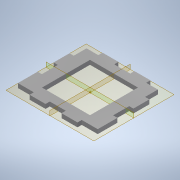
# Autodesk Inventor part: Plaat achter
Saved by Autodesk Inventor 2021 (Build 250183000, 183)
## iProperties
Manager: PJ / DCS
Company: Emmaüs Bovenbouw Aalter
Created: 2021-01-09
Part Number: Plaat achter
Material: S235
Catalog Web Link: http://emmausbovenbouw.op-weg.be/
Vendor: Emmaüsinstituut Bovenbouw Aalter
Document SubType Name: Modeling
Designer: Antho
Engineer: Declercq St.
Manufacturer: Standard
Standards Organization: Custom
Density: 7.86 g/cm^3
Appearance: Steel
Title: Algemene titel
Subject: Specifieke titel
Author: Antho
Keywords: Ruwe Ø xxxxx
Comments: Opmerking
Autodesk Inventor part; units mm, degrees
sketch "Sketch1" plane through (0, 0, 0) normal (0, 0, 1) x (1, 0, 0)
  line L0 (0, 2.8582) -> (0, -2.8582) construction
  line L1 (-5.7775, 0) -> (5.7775, 0) construction
  line L2 (-75, -68.5) -> (75, -68.5)
  line L3 (75, -68.5) -> (75, 68.5)
  line L4 (75, 68.5) -> (-75, 68.5)
  line L5 (-75, 68.5) -> (-75, -68.5)
  line L6 (-75, -68.5) -> (75, 68.5) construction
  line L7 (75, -68.5) -> (-75, 68.5) construction
  point P0 (0, 0)
  point P1 (0, 0)
  dimension "d0" = 150
  dimension "d1" = 137
  constraints: 16 end point, 4 midpoint, 2 horizontal, 2 parallel, 1 coincident, 1 perpendicular, 1 vertical
  measures "d0" distance of L4.end L3.end
  measures "d1" distance of L3.end L2.end
extrude "Extrusion1" add sketch "Sketch1" along normal blind 8
sketch "Sketch2" plane through (0, 0, 8) normal (0, 0, 1) x (1, 0, 0)
  line L0 (-75, -68.5) -> (75, -68.5) projected
  line L1 (0, -68.5) -> (-15, -68.5)
  line L2 (-15, -68.5) -> (15, -68.5)
  line L3 (15, -68.5) -> (45, -68.5)
  line L4 (-15, -68.5) -> (-45, -68.5)
  line L5 (-15, -68.5) -> (15, -68.5)
  line L6 (15, -68.5) -> (15, -60.5)
  line L7 (15, -60.5) -> (-15, -60.5)
  line L8 (-15, -60.5) -> (-15, -68.5)
  line L9 (75, -68.5) -> (75, 68.5) projected
  line L10 (45, -68.5) -> (75, -68.5)
  line L11 (75, -68.5) -> (75, -60.5)
  line L12 (75, -60.5) -> (45, -60.5)
  line L13 (45, -60.5) -> (45, -68.5)
  line L14 (-75, 68.5) -> (-75, -68.5) projected
  line L15 (-45, -68.5) -> (-75, -68.5)
  line L16 (-75, -68.5) -> (-75, -60.5)
  line L17 (-75, -60.5) -> (-45, -60.5)
  line L18 (-45, -60.5) -> (-45, -68.5)
  line L19 (75, -68.5) -> (75, -53.5)
  line L20 (75, -53.5) -> (75, -23.5)
  line L21 (75, -23.5) -> (75, 6.5)
  line L22 (75, 6.5) -> (75, 36.5)
  line L23 (75, 36.5) -> (75, 66.5)
  line L24 (75, -23.5) -> (67, -23.5)
  line L25 (67, -23.5) -> (67, 6.5)
  line L26 (67, 6.5) -> (75, 6.5)
  line L27 (75, 6.5) -> (75, -23.5)
  line L28 (75, 68.5) -> (-75, 68.5) projected
  line L29 (75, 36.5) -> (67, 36.5)
  line L30 (67, 36.5) -> (67, 68.5)
  line L31 (67, 68.5) -> (75, 68.5)
  line L32 (75, 68.5) -> (75, 36.5)
  line L33 (-75, -23.5) -> (-67, -23.5)
  line L34 (-67, -23.5) -> (-67, 6.5)
  line L35 (-67, 6.5) -> (-75, 6.5)
  line L36 (-75, 6.5) -> (-75, -23.5)
  line L37 (-75, 36.5) -> (-67, 36.5)
  line L38 (-67, 36.5) -> (-67, 68.5)
  line L39 (-67, 68.5) -> (-75, 68.5)
  line L40 (-75, 68.5) -> (-75, 36.5)
  line L41 (0, 68.5) -> (-15, 68.5)
  line L42 (-15, 68.5) -> (15, 68.5)
  line L43 (15, 68.5) -> (45, 68.5)
  line L44 (-15, 68.5) -> (-45, 68.5)
  line L45 (-75, 68.5) -> (-45, 68.5)
  line L46 (-45, 68.5) -> (-45, 60.5)
  line L47 (-45, 60.5) -> (-75, 60.5)
  line L48 (-75, 60.5) -> (-75, 68.5)
  line L49 (-15, 68.5) -> (15, 68.5)
  line L50 (15, 68.5) -> (15, 60.5)
  line L51 (15, 60.5) -> (-15, 60.5)
  line L52 (-15, 60.5) -> (-15, 68.5)
  line L53 (45, 68.5) -> (75, 68.5)
  line L54 (75, 68.5) -> (75, 60.5)
  line L55 (75, 60.5) -> (45, 60.5)
  line L56 (45, 60.5) -> (45, 68.5)
  point P0 (0, 0)
  point P1 (67, 60.5)
  point P2 (-67, 60.5)
  dimension "d4" = 15
  dimension "d5" = 30
  dimension "d6" = 30
  dimension "d7" = 30
  dimension "d8" = 30
  dimension "d9" = 8
  dimension "d10" = 15
  dimension "d11" = 30
  dimension "d12" = 30
  dimension "d13" = 30
  dimension "d14" = 30
  dimension "d15" = 8
  dimension "d16" = 8
  dimension "d17" = 8
  dimension "d24" = 15
  dimension "d25" = 30
  dimension "d26" = 30
  dimension "d27" = 30
  dimension "d28" = 8
  constraints: 106 end point, 28 point on line, 20 parallel, 10 horizontal, 10 perpendicular, 2 midpoint
  measures "d4" distance of L1.start L1.end
  measures "d5" distance of L1.end L2.end
  measures "d6" distance of L2.end L3.end
  measures "d7" distance of L1.end L4.end
  measures "d8" distance of L7.end L6.end
  measures "d9" distance of L6.end L5.end
  measures "d10" distance of L10.end L19.end
  measures "d11" distance of L19.end L20.end
  measures "d12" distance of L20.end L21.end
  measures "d13" distance of L21.end L22.end
  measures "d14" distance of L22.end L23.end
  measures "d15" distance of L25.end L26.end
  measures "d16" distance of L30.end L31.end
  measures "d17" distance of L35.end L34.end
  measures "d24" distance of L41.start L41.end
  measures "d25" distance of L41.end L42.end
  measures "d26" distance of L42.end L43.end
  measures "d27" distance of L41.end L44.end
  measures "d28" distance of L45.end L46.end
extrude "Extrusion2" cut sketch "Sketch2" against normal blind 8 contours L14 L17 L18 L0 | L8 L7 L6 L0 | L14 L35 L34 L33 | L14 L47 L38 L37 | L13 L12 L9 L0 | L14 L28 L38 L47 | L38 L28 L46 L47 | L24 L25 L26 L9 | L28 L50 L51 L52 | L29 L30 L55 L9 | L55 L30 L28 L9 | L28 L30 L55 L56
sketch "Sketch3" plane through (0, 0, 8) normal (0, 0, 1) x (1, 0, 0)
  line L0 (-45, -45) -> (45, -45)
  line L1 (45, -45) -> (45, 45)
  line L2 (45, 45) -> (-45, 45)
  line L3 (-45, 45) -> (-45, -45)
  line L4 (-45, -45) -> (45, 45) construction
  line L5 (45, -45) -> (-45, 45) construction
  point P0 (0, 0)
  dimension "d20" = 90
  dimension "d21" = 90
  constraints: 12 end point, 2 midpoint, 2 parallel, 1 horizontal, 1 perpendicular
  measures "d20" distance of L2.end L1.end
  measures "d21" distance of L1.end L0.end
extrude "Extrusion3" cut sketch "Sketch3" against normal blind 8
body "Solid1"
